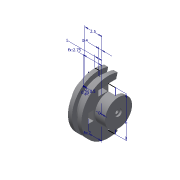
# Autodesk Inventor part: Gear platform_xw
Saved by Autodesk Inventor 2016 (Build 200138000, 138)
## iProperties
Created: 2014-06-19
Part Number: Gear platform_xw
Document SubType Name: Modeling
Designer: 121767
Density: 1 g/cm^3
Material: Generic
Appearance: Default
Author: 121767
Autodesk Inventor part; units mm, degrees
ref_plane "YZ Plane" through (0, 0, 0) normal (1, 0, 0) x (0, 1, 0)
ref_plane "XZ Plane" through (0, 0, 0) normal (0, 1, 0) x (-1, 0, 0)
sketch "Sketch1" plane through (0, 0, 0) normal (0, 0, 1) x (1, 0, 0)
  line L0 (-2.5, 1) -> (-2.5, 2)
  line L1 (-2.5, 2) -> (-1, 2)
  line L2 (-1, 2) -> (-1, 4)
  line L3 (-1, 4) -> (-0.4, 4)
  line L4 (-0.4, 4) -> (-0.4, 3.3)
  line L5 (-0.4, 3.3) -> (0, 3.3)
  line L6 (2, 2) -> (2, 0)
  line L7 (-2, 3) -> (-2, -3)
  line L8 (-2, -3) -> (2, -3)
  line L9 (-2, 3) -> (2, 3)
  line L10 (2, 3) -> (2, -3)
  line L11 (0, -5.1517) -> (0, 5.7378) construction
  line L12 (-2.5, 1) -> (-2.75, 1) construction
  line L13 (-2.75, 1) -> (-2.75, 0.75) construction
  line L14 (-2.75, 0.75) -> (-2.75, 0.5) construction
  line L15 (-2.75, 0.5) -> (-2.5, 0.5) construction
  line L16 (-2.25, 0.5) -> (-2.25, 0.25)
  line L17 (0, 3.3) -> (0, 0)
  line L18 (-2.25, 0.25) -> (-2, 0.25)
  line L19 (-2, 0) -> (0, 0)
  line L20 (-2.5, 1) -> (-2.5, 0.5)
  line L21 (-2.5, 0.5) -> (-2.25, 0.5)
  line L22 (-2, 0.25) -> (0, 0.25)
  dimension "d12" = 6
  dimension "d49" = 2
  dimension "d50" = 2.5
  dimension "d51" = 1
  dimension "d52" = 0.4
  dimension "d54" = 2.75
  dimension "d62" = 0.5
  dimension "d64" = 0
  dimension "d67" = 0.25
  constraints: 46 end point, 8 perpendicular, 5 point on line, 4 parallel, 1 collinear, 1 horizontal, 1 midpoint, 1 other
  measures "d12" distance between parallel lines of L8 L9
  measures "d49" distance between parallel lines of L7 L11
  measures "d50" distance between parallel lines of L11 L0
  measures "d51" distance between parallel lines of L2 L11
  measures "d52" distance between parallel lines of L11 L4
  measures "d54" distance between parallel lines of L13 L11
  measures "d62" distance of L14.end L16.start
  measures "d64" distance of L17.end point (0, 0)
  measures "d67" distance between parallel lines of L19 L18
revolve "Revolution1" add sketch "Sketch1" angle 360 about axis through (-2, 0, 0) along (1, 0, 0) contours L0 L1 L7 L18 L16 L21 L20 | L1 L2 L9 L17 L22 L7 | L22 L17 L19 L7 | L2 L3 L4 L5 L17 L9
mirror "Mirror1" about plane through (0, 0, 0) normal (1, 0, 0) of "Revolution1"
extrude "Extrusion1" cut sketch "Sketch1" against normal blind 25.4 contours L7 L9 L2 L1 | L1 L2 L9 L17 L22 L7 | L22 L17 L19 L7 | L19 L17 L9 L10 L6 L8 L7
hole "Hole3" [suppressed]
chamfer "Chamfer1" distance 1.5 angle 45 2 edges at (-0.7, -3, -2.6458) (-0.7, 3, -2.6458)
pattern_of_nothing "Mirror2"
hole "Hole4" at (2, 0, 0) direction (-1, 0, 0) diameter 1 depth 4
ref_plane "Work Plane5" through (1, 0, 0) normal (1, 0, 0) x (0, 0, -1)
sketch "Sketch6" plane through (1, 0, 0) normal (1, 0, 0) x (0, 0, -1)
  arc A0 (0, 2) -> (0, -2) centre (0, 0) ccw projected
  line L0 (-3, 0.7) -> (-2.2, 0.7)
  line L1 (-2.2, 0.7) -> (-2.2, -0.7)
  line L2 (-2.2, -0.7) -> (-3, -0.7)
  line L3 (-3, -0.7) -> (-3, 0.7)
  arc A1 (1.1693, 3.0859) -> (1.1693, -3.0859) centre (0, 0) ccw projected
  line L4 (-0.1, 2.08) -> (-1.5, 2.08)
  line L5 (-1.5, 2.08) -> (-1.5, 2.88)
  line L6 (-1.5, 2.88) -> (-0.1, 2.88)
  line L7 (-0.1, 2.88) -> (-0.1, 2.08)
  line L8 (0, 3) -> (0, 2) projected
  point P0 (-2.2, 0)
  dimension "d101" = 0.8
  dimension "d102" = 1.4
  dimension "d103" = 2.2
  dimension "d104" = 1.4
  dimension "d105" = 0.8
  dimension "d106" = 0.1
  dimension "d107" = 0.08
  constraints: 16 end point, 4 parallel, 2 horizontal, 2 perpendicular, 1 horizontal alignment, 1 midpoint
  measures "d101" distance of L0.start L0.end
  measures "d102" distance of L2.end L0.start
  measures "d103" distance from line of point (0, 0) L1
  measures "d104" distance of L5.end L6.end
  measures "d105" distance of L4.end L5.end
  measures "d106" distance between parallel lines of L8 L7
  measures "d107" distance from line of L8.end L4
extrude "Extrusion6" cut sketch "Sketch6" against normal blind 1.8
ref_plane "Work Plane1" through (0, 0, 0) normal (1, 0, 0) x (0, 1, 0)
body "Solid1"
